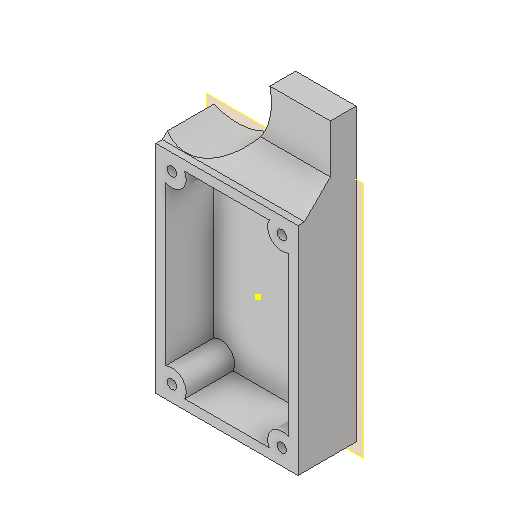
# Autodesk Inventor part: cellSTORM_v5_cellphone_craddle
Saved by Autodesk Inventor 2022 (Build 260153000, 153)
## iProperties
Created: 2021-08-26
Part Number: cellSTORM_v5_cellphone_craddle
Material: Generic
Document SubType Name: Modeling
Designer: diederichbenedict
Density: 1 g/cm^3
Appearance: Default
Author: diederichbenedict
Autodesk Inventor part; units mm, degrees
ref_plane "YZ Plane" through (0, 0, 0) normal (1, 0, 0) x (0, 1, 0)
ref_plane "XZ Plane" through (0, 0, 0) normal (0, 1, 0) x (-1, 0, 0)
sketch "Sketch1" plane through (0, 0, 0) normal (0, 0, 1) x (1, 0, 0)
  circle A0 centre (7.3112, -36.65) radius 1.4 projected
  circle A1 centre (-26.6888, 20.35) radius 1.4 projected
  circle A2 centre (7.3112, 20.35) radius 1.4 projected
  circle A3 centre (-26.6888, -36.65) radius 1.4 projected
  line L0 (12.3112, -41.65) -> (12.3112, 25.35) projected
  line L1 (12.3112, -41.65) -> (-31.6888, -41.65) projected
  line L2 (-31.6888, -41.65) -> (-31.6888, 25.35) projected
  line L3 (12.3112, 25.35) -> (-31.6888, 25.35) projected
  point P0 (0, 0)
ref_plane "Work Plane1" through (0, 0, -18) normal (0, 0, 1) x (1, 0, 0)
sketch "Sketch2" plane through (0, 0, -18) normal (0, 0, 1) x (1, 0, 0)
  circle A0 centre (-24.44, 44) radius 15.35 projected
  circle A1 centre (7.3112, -36.65) radius 1.4 projected
  circle A2 centre (-26.6888, 20.35) radius 1.4 projected
  circle A3 centre (7.3112, 20.35) radius 1.4 projected
  circle A4 centre (-26.6888, -36.65) radius 1.4 projected
  line L0 (12.3112, -41.65) -> (12.3112, 25.35) projected
  line L1 (12.3112, -41.65) -> (-31.6888, -41.65) projected
  line L2 (-31.6888, -41.65) -> (-31.6888, 25.35) projected
  line L3 (12.3112, 25.35) -> (-31.6888, 25.35) projected
  line L4 (12.3112, -41.65) -> (-31.6888, -41.65)
  line L5 (-31.6888, -41.65) -> (-31.6888, 26.9137)
  line L6 (12.3112, 48.35) -> (12.3112, -41.65)
  circle A5 centre (-24.44, 44) radius 15.35 projected
  arc A6 (-31.8604, 26.9875) -> (-6.3966, 48.35) centre (-24.44, 44) ccw
  line L7 (-31.6888, 48.35) -> (-9.7193, 48.35)
  line L8 (-6.3966, 48.35) -> (12.3112, 48.35)
  point P0 (0, 0)
  dimension "d1" = 90
  constraints: 10 end point, 3 parallel, 3 point on circle, 1 centre point, 1 coincident, 1 horizontal, 1 perpendicular, 2 other
  measures "d1" distance of L4.end L7.start
extrude "Extrusion1" add sketch "Sketch1" against normal blind 10
extrude "Extrusion2" add sketch "Sketch2" along normal up to surface (8 mm away) contours L1 L2 L3 L0 | L3 L5 A6 L8 L6
chamfer "Chamfer1" distance 8 angle 45 1 edges at (-9.6888, 25.35, -10)
sketch "Sketch3" plane through (0, 0, 0) normal (0, 0, 1) x (1, 0, 0)
  point P0 (0, 0)
shell "Shell1" thickness 3 removed faces 1 at (-4.2872, -17.2659, 0)
sketch "Sketch4" plane through (0, 0, -18) normal (0, 0, -1) x (-1, 0, 0)
  circle A0 centre (26.6888, -36.65) radius 1.4 projected
  circle A1 centre (-7.3112, 20.35) radius 1.4 projected
  circle A2 centre (26.6888, 20.35) radius 1.4 projected
  circle A3 centre (-7.3112, -36.65) radius 1.4 projected
  line L0 (-12.3112, -41.65) -> (31.6888, -41.65) projected
  line L1 (31.6888, -41.65) -> (31.6888, 26.9137) projected
  arc A4 (6.3966, 48.35) -> (31.6888, 26.9137) centre (24.44, 44) ccw projected
  line L2 (6.3966, 48.35) -> (-12.3112, 48.35) projected
  line L3 (-12.3112, 48.35) -> (-12.3112, -41.65) projected
  line L4 (8.9105, 5.35) -> (8.9105, 25.35)
  point P0 (0, 0)
  constraints: 2 end point, 1 vertical, 2 other
hole "Hole1" at (7.3112, 20.35, -18) at (-26.6888, 20.35, -18) at (-26.6888, -36.65, -18) at (7.3112, -36.65, -18) direction (0, 0, 1) diameter 2.9 end through all counterbore diameter 7 counterbore depth 4
body "Solid1"
